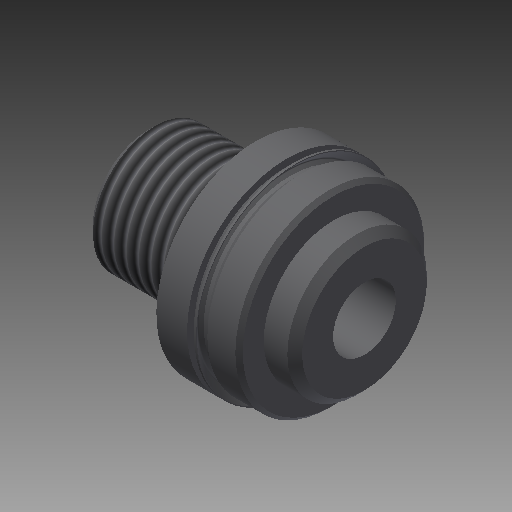
# Autodesk Inventor part: 04000-0_rod_guide
Saved by Autodesk Inventor 2017 (Build 210142000, 142)
## iProperties
Category: PARTsolutions
Company: BIMBA
Created: 2016-10-01
Part Number: 04000-0_rod_guide
Catalog Web Link: www.cadenas.de
Description: Rod Guide-Original Line - Standard Air Cylinders
Vendor: BIMBA
Document SubType Name: Modeling
Designer: psAdmin
Manufacturer: BIMBA
Mass: 3.5706 g
Surface Area: 22.4703 cm^2
Volume: 3.5706 cm^3
Density: 1 g/cm^3
Material: Generic
Appearance: PSOLRGB-211-211-211
PSOL_IDENT_0: {$CADENAS_DATA\23d-libs\bimba\bimba\bimba_imperial\bimba_full_line\original_line_cylinders\standard_
PSOL_IDENT_1: air_cylinders\rod_guide.prj},230 {VTYP=3D},{NB=04000-0_rod_guide},{LINA=04000-0_rod_guide},{NN=Rod G
PSOL_IDENT_2: uide},{DATE=22.09.2016 13:52:24},{GEOMDATE=07.11.2015 13:30:00},{VERSION=},{LINEID=40},{LINESUBID=-1
PSOL_IDENT_3: },{WBVAR=MNT,ACTING,NR,K,Q,T1,T2,T3,T4,MB,TRIM,CUSH,RODTRANS}  {NB=04000-0_rod_guide},{LINA=04000-0_
PSOL_IDENT_4: rod_guide},{KT=DUMMY},{PN=04000},{BORE=0.75000000},{BOREPN=04},{MNT=},{MNTALG='' , 'Front Nose' , 'B
PSOL_IDENT_5: F' , 'Front Block' , 'BFT' , 'Front Trunnion' , 'A' , 'Adjustable Stroke'},{ACTING=},{ACTINGALG= ''
PSOL_IDENT_6: , 'Single Acting' , 'R' , 'Reverse/Double Acting' },{NR=},{NRALG= '' , 'Without Non-rotating Rod' , '
PSOL_IDENT_7: NR' , 'With Non-rotating Rod' },{K=},{Q=},{QALG= '' , 'Without Side Ported Rear Head' , 'Q' , 'With
PSOL_IDENT_8: Side Ported Rear Head' },{T1=},{T2=},{T3=},{T4=},{MB=0},{A1=0.8750},{A1N=0.8750},{A1P=1.5940},{A1B=1
PSOL_IDENT_9: .5940},{A2=0.4380},{A2N=0.4380},{A2P=0.5000},{A3=0.1240},{A3N=0.1240},{A3P=0.8440},{A4=0.3130},{A4N=
PSOL_IDENT_10: 0.3130},{A4P=0.2525},{A5=0.0300},{A6=0.1250},{A6N=0.1250},{A6P=0.0000},{A7=0.4390},{A7N=0.4390},{A7P=
PSOL_IDENT_11: 0.2500},{A8=0.0100},{A8N=0.0100},{A8NR=0.0300},{D1=0.8050},{D1N=0.8050},{D1P=0.8625},{D1B=0.8325},{D
PSOL_IDENT_12: 2=0.7615},{D3=0.5620},{D3N=0.5620},{D3P=0.0000},{D4=0.2605},{D4N=0.2605},{D4P=0.5310},{D4NR=0.3120},
PSOL_IDENT_13: {D5=0.2535},{D5N=0.2535},{D5NR=0.2515},{C1=0.030},{C2=0.0150},{C2N=0.0150},{C2P=0.0300},{C3=0.0000},
PSOL_IDENT_14: {C3N=0.0000},{C3P=0.0000},{C4=0.0000},{C4N=0.0000},{C4P=0.0300},{NDM=0.5000},{NDMN=0.5000},{NDMP=0.6
PSOL_IDENT_15: 250},{TAB=UNF},{D6=0.6225},{D6N=0.6225},{D6P=0.6225},{A9=0.0940},{A9N=0.0940},{A9P=0.0940},{D7=0.538
PSOL_IDENT_16: 5},{D7N=0.5385},{D7P=0.5385},{A10=0.0855},{A10N=0.0855},{A10P=0.0855},{R1=0.0345},{R1N=0.0345},{R1P=
PSOL_IDENT_17: 0.0345},{D8=0.5310},{D9=0.5000},{D10=0.4405},{A11=0.8030},{A12=0.8970},{A13=1.0220},{A14=0.6250},{A1
PSOL_IDENT_18: 4N=0.6250},{A14B=0.6250},{D11=0.2500},{D11N=0.2500},{NDM2=0.4050},{NDM2N=0.4050},{NDM2DP=0.2500},{TH
PSOL_IDENT_19: READ=1},{HEX=0.2535},{HEXN=0.2535},{S1=1.0000},{B1=0.1250},{B2=0.4690},{B22=0.0000},{DB=0.0000},{B3=
PSOL_IDENT_20: 0.3800},{B4=0.6300},{X1=0.0920},{X2=0.6225},{NDM3=0.2500},{NDM4=0.1900},{NDM4DP=0.2500},{DD=1.0000},
PSOL_IDENT_21: {CB=0.3280},{CBDP=0.2190},{PORT=1},{XT=0.4380},{XTX=0.4380},{XT1=0.5000},{XT2=0.3750},{NDMH=0.4375},
PSOL_IDENT_22: {OD=0.8050},{ID=0.7615},{G=0.0000},{PNUT=0.4380},{TRIM=0},{C11=0.2380},{C22=0.2750},{C33=0.1950},{C4
PSOL_IDENT_23: 4=0.3700},{C55=0.5350},{CD1=0.1900},{CD2=0.1500},{CD3=0.0725},{CNDM3=0.1380},{CTAB3=UNF},{CUSH=0},{X
PSOL_IDENT_24: X=0.63000},{LCD=0.0000},{RODTRANS=0.00000}
NN: Rod Guide
NT: Original Line - Standard Air Cylinders
NB: 04000-0_rod_guide
NBSYN: $PN.-$RODTRANS._rod_guide
LINA: 04000-0_rod_guide
BORE: 3/4
BOREPN: 04
MNT: Front Nose
MNTALG: '' , 'Front Nose' , 'BF' , 'Front Block' , 'BFT' , 'Front Trunnion' , 'A' , 'Adjustable Stroke'
ACTING: Single Acting
NR: Without Non-rotating Rod
K: Standard
Q: Without Side Ported Rear Head
T1: without T1
T2: without T2
T3: without T3
T4: without T4
MB: 0
A1N: 0.8750
A1P: 1.5940
A1B: 1.5940
A2N: 0.4380
A2P: 0.5000
A3N: 0.1240
A3P: 0.8440
A4N: 0.3130
A4P: 0.2525
A5: 0.0300
A6N: 0.1250
A6P: 0.0000
A7N: 0.4390
A7P: 0.2500
A8N: 0.0100
A8NR: 0.0300
D1N: 0.8050
D1P: 0.8625
D1B: 0.8325
D2: 0.7615
D3N: 0.5620
D3P: 0.0000
D4N: 0.2605
D4P: 0.5310
D4NR: 0.3120
D5N: 0.2535
D5NR: 0.2515
C1: 0.030
C2N: 0.0150
C2P: 0.0300
C3N: 0.0000
C3P: 0.0000
C4N: 0.0000
C4P: 0.0300
NDMN: 0.5000
NDMP: 0.6250
TAB: UNF
D6N: 0.6225
D6P: 0.6225
A9N: 0.0940
A9P: 0.0940
D7N: 0.5385
D7P: 0.5385
A10N: 0.0855
A10P: 0.0855
R1N: 0.0345
R1P: 0.0345
D8: 0.5310
D9: 0.5000
D10: 0.4405
A11: 0.8030
A12: 0.8970
A13: 1.0220
A14N: 0.6250
A14B: 0.6250
D11N: 0.2500
NDM2N: 0.4050
NDM2DP: 0.2500
HEXN: 0.2535
S1: 1.0000
B1: 0.1250
B2: 0.4690
B22: 0.0000
DB: 0.0000
B3: 0.3800
B4: 0.6300
X1: 0.0920
X2: 0.6225
NDM3: 0.2500
NDM4: 0.1900
NDM4DP: 0.2500
DD: 1.0000
CB: 0.3280
CBDP: 0.2190
XTX: 0.4380
XT1: 0.5000
XT2: 0.3750
NDMH: 0.4375
TRIM: 0
C11: 0.2380
C22: 0.2750
C33: 0.1950
C44: 0.3700
C55: 0.5350
CD1: 0.1900
CD2: 0.1500
CD3: 0.0725
CNDM3: 0.1380
CTAB3: UNF
CUSH: 0
LCD: 0.0000
RODTRANS: 0.00000
SUPPLIER: BIMBA
ARTICLENO: 04000-0_rod_guide
BOMINFO: 04000-0_rod_guide
CREATOR: CADENAS GmbH
Title: 04000-0_rod_guide
Author: Cadenas PARTsolutions
Comments: Original Line - Standard Air Cylinders
Autodesk Inventor part; units mm, degrees
ref_plane "YZ Plane" through (0, 0, 0) normal (1, 0, 0) x (0, 1, 0)
ref_plane "XZ Plane" through (0, 0, 0) normal (0, 1, 0) x (-1, 0, 0)
ref_plane "XY Plane" through (0, 0, 0) normal (0, 0, 1) x (1, 0, 0)
sketch "Sketch_1" plane through (0, 0, 0) normal (0, 0, 1) x (1, 0, 0)
  line L0 (11.1252, 0) -> (0, 0)
  line L1 (0, 0) -> (0, 5.5944)
  line L2 (0, 5.5944) -> (0.7557, 6.35)
  line L3 (0.7557, 6.35) -> (11.1252, 6.35)
  line L4 (11.1252, 6.35) -> (11.1252, 0)
  line L5 (11.1252, 0) -> (0, 0)
  constraints: 12 end point
revolve "Revolution1" add sketch "Sketch_1" angle 360 about axis through (11.1252, 0, 0) along (1, 0, 0)
thread "Thread1" size "1/2-20 UNF" class "2A" standard "ANSI Unified Screw Threads" full length
sketch "Sketch_3" plane through (0, 0, 0) normal (0, 0, 1) x (1, 0, 0)
  line L0 (19.05, 0) -> (11.1252, 0)
  line L1 (11.1252, 0) -> (11.1252, 10.2235)
  line L2 (11.1252, 10.2235) -> (14.2748, 10.2235)
  line L3 (14.2748, 10.2235) -> (14.2748, 8.9091)
  line L4 (14.2748, 8.9091) -> (15.0368, 8.9091)
  line L5 (15.0368, 8.9091) -> (15.7988, 9.671)
  line L6 (15.7988, 9.671) -> (18.669, 9.671)
  line L7 (18.669, 9.671) -> (19.05, 9.2901)
  line L8 (19.05, 9.2901) -> (19.05, 0)
  line L9 (19.05, 0) -> (11.1252, 0)
  constraints: 20 end point
revolve "Revolution2" add sketch "Sketch_3" angle 360 about axis through (19.05, 0, 0) along (1, 0, 0)
sketch "Sketch_4" plane through (0, 0, 0) normal (0, 0, 1) x (1, 0, 0)
  line L0 (22.225, 0) -> (19.05, 0)
  line L1 (19.05, 0) -> (19.05, 7.1374)
  line L2 (19.05, 7.1374) -> (21.463, 7.1374)
  line L3 (21.463, 7.1374) -> (22.225, 6.3754)
  line L4 (22.225, 6.3754) -> (22.225, 0)
  line L5 (22.225, 0) -> (19.05, 0)
  constraints: 12 end point
revolve "Revolution3" add sketch "Sketch_4" angle 360 about axis through (22.225, 0, 0) along (1, 0, 0)
sketch "Sketch4" plane through (0, 0, 0) normal (-1, 0, 0) x (0, 0, 1)
  point P0 (0, 0)
hole "Hole1" at (0, 0, 0) direction (1, 0, 0) diameter 6.4389 depth 22.225 countersink diameter 6.9469 countersink angle 90
sketch "Sketch_47" plane through (0, 0, 0) normal (0, 0, 1) x (1, 0, 0)
  line L0 (15.0368, 0) -> (14.2748, 0)
  line L1 (14.2748, 9.512) -> (14.2748, 8.655)
  line L2 (14.2748, 8.655) -> (15.0368, 8.655)
  line L3 (15.0368, 8.655) -> (15.0368, 8.9091)
  line L4 (15.0368, 8.9091) -> (14.6558, 8.9091)
  line L5 (14.6558, 8.9091) -> (14.3973, 9.1676)
  arc A0 (14.3973, 9.3472) -> (14.3973, 9.1676) centre (14.4871, 9.2574) ccw
  line L6 (14.3973, 9.3472) -> (15.1895, 10.1393)
  line L7 (15.1895, 10.1393) -> (15.1895, 10.2235)
  line L8 (15.1895, 10.2235) -> (14.9863, 10.2235)
  line L9 (14.9863, 10.2235) -> (14.2748, 9.512)
  constraints: 20 end point, 2 point on circle, 1 centre point
revolve "Revolution4" add sketch "Sketch_47" angle 360 about axis through (15.0368, 0, 0) along (1, 0, 0)
ref_plane "hh_XY" through (0, 6.35, 0) normal (0, 0, 1) x (1, 0, 0)
ref_plane "hh_YZ" through (0, 6.35, 0) normal (1, 0, 0) x (0, 1, 0)
ref_plane "hh_ZX" through (0, 6.35, 0) normal (0, 1, 0) x (0, 0, 1)
ref_plane "rod_guide_XY" through (0, 0, 0) normal (1, 0, 0) x (0, 0, -1)
ref_plane "rod_guide_YZ" through (0, 0, 0) normal (0, 0, -1) x (0, 1, 0)
ref_plane "rod_guide_ZX" through (0, 0, 0) normal (0, 1, 0) x (1, 0, 0)
ref_plane "t1_XY" through (11.1252, 0, 0) normal (1, 0, 0) x (0, 0, -1)
ref_plane "t1_YZ" through (11.1252, 0, 0) normal (0, 0, -1) x (0, 1, 0)
ref_plane "t1_ZX" through (11.1252, 0, 0) normal (0, 1, 0) x (1, 0, 0)
ref_plane "t111_XY" through (11.1252, 0, 0) normal (1, 0, 0) x (0, 0, -1)
ref_plane "t111_YZ" through (11.1252, 0, 0) normal (0, 0, -1) x (0, 1, 0)
ref_plane "t111_ZX" through (11.1252, 0, 0) normal (0, 1, 0) x (1, 0, 0)
ref_plane "to_foot_bracket_XY" through (11.1252, 0, 0) normal (1, 0, 0) x (0, 0, -1)
ref_plane "to_foot_bracket_YZ" through (11.1252, 0, 0) normal (0, 0, -1) x (0, 1, 0)
ref_plane "to_foot_bracket_ZX" through (11.1252, 0, 0) normal (0, 1, 0) x (1, 0, 0)
ref_plane "to_nut_XY" through (11.1252, 0, 0) normal (1, 0, 0) x (0, 0, -1)
ref_plane "to_nut_YZ" through (11.1252, 0, 0) normal (0, 0, -1) x (0, 1, 0)
ref_plane "to_nut_ZX" through (11.1252, 0, 0) normal (0, 1, 0) x (1, 0, 0)
ref_plane "to_rod_XY" through (0, 0, 0) normal (1, 0, 0) x (0, 0, -1)
ref_plane "to_rod_YZ" through (0, 0, 0) normal (0, 0, -1) x (0, 1, 0)
ref_plane "to_rod_ZX" through (0, 0, 0) normal (0, 1, 0) x (1, 0, 0)
ref_plane "to_screw_XY" through (6.35, 2.032, -6.0452) normal (0, 1, 0) x (1, 0, 0)
ref_plane "to_screw_YZ" through (6.35, 2.032, -6.0452) normal (1, 0, 0) x (0, 0, -1)
ref_plane "to_screw_ZX" through (6.35, 2.032, -6.0452) normal (0, 0, -1) x (0, 1, 0)
ref_plane "to_trunnion_brackets_XY" through (11.1252, 0, 0) normal (0, 1, 0) x (1, 0, 0)
ref_plane "to_trunnion_brackets_YZ" through (11.1252, 0, 0) normal (1, 0, 0) x (0, 0, -1)
ref_plane "to_trunnion_brackets_ZX" through (11.1252, 0, 0) normal (0, 0, -1) x (0, 1, 0)
ref_plane "to_trunnion_brackets1_XY" through (11.1252, 12.7, 0) normal (0, 1, 0) x (1, 0, 0)
ref_plane "to_trunnion_brackets1_YZ" through (11.1252, 12.7, 0) normal (1, 0, 0) x (0, 0, -1)
ref_plane "to_trunnion_brackets1_ZX" through (11.1252, 12.7, 0) normal (0, 0, -1) x (0, 1, 0)
ref_plane "to_trunnion_brackets2_XY" through (11.1252, -12.7, 0) normal (0, 1, 0) x (1, 0, 0)
ref_plane "to_trunnion_brackets2_YZ" through (11.1252, -12.7, 0) normal (1, 0, 0) x (0, 0, -1)
ref_plane "to_trunnion_brackets2_ZX" through (11.1252, -12.7, 0) normal (0, 0, -1) x (0, 1, 0)
ref_plane "to_tube_XY" through (15.0368, 0, 0) normal (1, 0, 0) x (0, 0, -1)
ref_plane "to_tube_YZ" through (15.0368, 0, 0) normal (0, 0, -1) x (0, 1, 0)
ref_plane "to_tube_ZX" through (15.0368, 0, 0) normal (0, 1, 0) x (1, 0, 0)
body "Solid1"
